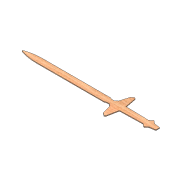
# Autodesk Inventor part: Romeo And Juliette Sword
Saved by Autodesk Inventor 2021 (Build 250183000, 183)
## iProperties
Created: 2018-05-23
Part Number: Romeo And Juliette Sword
Material: Wood (Birch)
Document SubType Name: Modeling
Designer: dbrui
Density: 0.55 g/cm^3
Appearance: Birch - Natural Polished
Author: dbrui
Autodesk Inventor part; units mm, degrees
ref_plane "YZ Plane" through (0, 0, 0) normal (1, 0, 0) x (0, 1, 0)
ref_plane "XZ Plane" through (0, 0, 0) normal (0, 1, 0) x (-1, 0, 0)
ref_plane "XY Plane" through (0, 0, 0) normal (0, 0, 1) x (1, 0, 0)
sketch "Sketch1" plane through (0, 0, 0) normal (0, 1, 0) x (-1, 0, 0)
  line L0 (457.2, 76.2) -> (-457.2, 76.2) construction
  line L1 (-457.2, 76.2) -> (-457.2, -76.2) construction
  line L2 (-457.2, -76.2) -> (457.2, -76.2) construction
  line L3 (457.2, -76.2) -> (457.2, 76.2) construction
  line L4 (457.2, 76.2) -> (-457.2, -76.2) construction
  line L5 (-457.2, 76.2) -> (457.2, -76.2) construction
  line L6 (-457.2, 7.9375) -> (-457.2, -7.9375)
  line L7 (-457.2, -7.9375) -> (-432.0472, -11.4725)
  line L8 (-457.2, -7.9375) -> (-431.8, -7.9375) construction
  line L9 (-457.2, 7.9375) -> (-432.0472, 11.4725)
  line L10 (-457.2, 7.9375) -> (-431.8, 7.9375) construction
  line L11 (-432.0472, 11.4725) -> (-432.0472, -11.4725)
  line L12 (-432.0472, 11.4725) -> (-419.3472, 21.8097)
  line L13 (-419.3472, 21.8097) -> (-419.3472, -21.8097)
  line L14 (-419.3472, -21.8097) -> (-432.0472, -11.4725)
  line L15 (-406.6472, 11.4725) -> (-406.6472, -11.4725)
  line L16 (-406.6472, 11.4725) -> (-419.3472, 21.8097)
  line L17 (-419.3472, -21.8097) -> (-406.6472, -11.4725)
  line L18 (-324.0972, 13.5255) -> (-324.0972, -13.5255)
  line L19 (-324.0972, 13.5255) -> (-406.6472, 11.4725)
  line L20 (-324.0972, -13.5255) -> (-406.6472, -11.4725)
  line L21 (-324.0972, 13.5255) -> (-298.6972, 13.5255) construction
  line L22 (-324.0972, -13.5255) -> (-298.6972, -13.5255) construction
  line L23 (-406.6472, 0) -> (-401.5952, 0)
  line L24 (44.2028, 13.5255) -> (44.2028, -13.5255)
  line L25 (-244.337, 13.5255) -> (44.2028, 13.5255)
  line L26 (44.2028, -13.5255) -> (-244.337, -13.5255)
  arc A0 (120.4028, 0) -> (44.2028, 13.5255) centre (44.2028, -207.8851) ccw
  arc A1 (44.2028, -13.5255) -> (120.4028, 0) centre (44.2028, 207.8851) ccw
  arc A2 (-244.337, -13.5255) -> (-254.0713, -10.3505) centre (-254.0713, -26.8605) ccw
  arc A3 (-254.0713, 10.3505) -> (-244.337, 13.5255) centre (-254.0713, 26.8605) ccw
  line L27 (-254.0713, -10.3505) -> (-269.9463, -10.3505)
  line L28 (-254.0713, 10.3505) -> (-269.9463, 10.3505)
  line L29 (-298.6947, -64.7889) -> (-285.8213, -64.7889)
  line L30 (-285.8213, -64.7889) -> (-269.9463, -10.3505)
  line L31 (-298.6947, 64.7889) -> (-285.8213, 64.7889)
  line L32 (-285.8213, 64.7889) -> (-269.9463, 10.3505)
  line L33 (-324.0972, -13.5255) -> (-318.7941, -13.5255)
  line L34 (-324.0972, 13.5255) -> (-318.7941, 13.5255)
  line L35 (-308.7454, -13.5255) -> (-298.6947, -64.7889)
  line L36 (-308.7454, 13.5255) -> (-298.6947, 64.7889)
  line L37 (-324.0972, -13.5255) -> (-308.7454, -13.5255)
  line L38 (-324.0972, 13.5255) -> (-308.7454, 13.5255)
  point P0 (0, 0)
  point P1 (-457.2, 0)
  point P2 (-457.2, 0)
  point P3 (44.2028, 0)
  point P4 (0, 0)
  point P5 (0, 0)
  dimension "d0" = 914.4
  dimension "d1" = 152.4
  dimension "d3" = 15.875
  dimension "d4" = 25.4
  dimension "d5" = 8
  dimension "d6" = 25.4
  dimension "d7" = 8
  dimension "d8" = 12.7
  dimension "d9" = 16.3752
  dimension "d10" = 16.3752
  dimension "d11" = 27.051
  dimension "d25" = 27.051
  dimension "d27" = 76.2
  dimension "d37" = 16.51
  dimension "d38" = 16.51
  dimension "d63" = 3.175
  dimension "d64" = 3.175
  dimension "d71" = 56.7059
  dimension "d72" = 56.7059
  dimension "d73" = 12.8734
  dimension "d74" = 12.8734
  dimension "d75" = 52.2394
  dimension "d76" = 52.2394
  dimension "d77" = 27.35
  dimension "d78" = 412.9972
  dimension "d79" = 256.2545
  dimension "d80" = 701.537
  dimension "d81" = 701.537
  dimension "d82" = 755.8972
  dimension "d83" = 755.8972
  dimension "d84" = 775.9941
  dimension "d85" = 775.9941
  dimension "d86" = 858.7952
  dimension "d87" = 16.257
  dimension "d88" = 88.575
  constraints: 78 end point, 10 horizontal, 8 midpoint, 8 point on circle, 6 horizontal alignment, 6 point on line, 4 centre point, 4 tangent, 4 vertical, 3 parallel, 3 symmetric about line, 2 coincident, 2 equal length, 1 perpendicular
  measures "d0" distance of L2.end L1.end
  measures "d1" distance of L1.end L0.end
  measures "d3" distance of L6.start L6.end
  measures "d4" distance of L6.end L7.end
  measures "d5" angle of L7 L8
  measures "d6" distance of L6.start L9.end
  measures "d7" angle of L10 L9
  measures "d8" horizontal distance of L9.end L12.end
  measures "d9" distance of L9.end L12.end
  measures "d10" distance of L13.end L7.end
  measures "d11" distance of L18.start L18.end
  measures "d25" distance of L24.start L24.end
  measures "d27" distance of point (44.203, 0) A0.start
  measures "d37" radius of A3
  measures "d38" radius of A2
  measures "d63" distance between parallel lines of L25 L28
  measures "d64" distance between parallel lines of L26 L27
  measures "d71" distance of L31.end L28.end
  measures "d72" distance of L29.end L27.end
  measures "d73" distance of L29.start L29.end
  measures "d74" distance of L31.start L31.end
  measures "d75" distance of L36.start L31.start
  measures "d76" distance of L35.start L29.start
  measures "d77" angle of L35 L30
  measures "d78" distance between parallel lines of L3 L24
  measures "d79" distance from line of point (0, 0) L32
  measures "d80" distance from line of L25.start L3
  measures "d81" distance from line of L26.end L3
  measures "d82" distance from line of L21.end L3
  measures "d83" distance from line of L22.end L3
  measures "d84" distance from line of L34.end L3
  measures "d85" distance from line of L33.end L3
  measures "d86" distance from line of L23.end L3
  measures "d87" angle of L32 L3
  measures "d88" angle of L19 L3
extrude "Extrusion4" add sketch "Sketch1" along normal blind 3.175
chamfer "Chamfer2" distance 3.175 angle 45 3 edges at (298.6947, 1.5875, 64.7889) (298.6947, 1.5875, -64.7889) (308.7454, 1.5875, 13.5255)
fillet "Fillet4" radius 1.651 11 edges at (254.0713, 1.5875, 10.3505) (254.0713, 1.5875, -10.3505) (-120.4028, 1.5875, 0) (457.2, 1.5875, 7.9375) (432.0472, 1.5875, 11.4725) (419.3472, 1.5875, 21.8097) (406.6472, 1.5875, 11.4725) (457.2, 1.5875, -7.9375) (419.3472, 1.5875, -21.8097) (432.0472, 1.5875, -11.4725) (406.6472, 1.5875, -11.4725)
fillet "Fillet6" radius 6.35 2 edges at (324.0972, 1.5875, 13.5255) (324.0972, 1.5875, -13.5255)
chamfer "Chamfer3" distance 7.9375 angle 45 4 edges at (269.9463, 1.5875, 10.3505) (285.8213, 1.5875, 64.7889) (285.8213, 1.5875, -64.7889) (269.9463, 1.5875, -10.3505)
equation "\"d4\" = d6"
equation "\"d7\" = d5"
equation "\"d10\" = d9"
equation "\"d25\" = d11"
equation "\"d38\" = d37"
equation "\"d64\" = d63"
body "Solid3"
